Autodesk Fusion 360 part; units mm, degrees
note: some values were not read from the file. Chosen so that the rebuilt part matches the saved one: which bodies a step acts on. Set by a fixed rule: which sketch regions a step uses.
(part 2 of 2)
  measures "d487" distance of P900 P901
  measures "d488" distance of P898 P900
  measures "d489" radius of A29
  measures "d490" distance of P902 L38
  measures "d491" distance of P902 L39
  measures "d492" horizontal distance of P899 P902
  measures "d493" vertical distance of P899 P902
  measures "d603" distance of L42.start L42.end
  measures "d604" distance of L42.end L43.end
  measures "d608" diameter of A30
extrude "Extruir23" cut sketch "Boceto5" against normal blind 5 contours L8 L9 L10 L13 | L8 L9 L12 L13 | L8 L9 L11 L12 | L8 L9 L10 L11 | L8 L12 L42 L43 | L8 L12 L44 L45 bodies 10
extrude "Extruir24" add sketch "Boceto5" against normal blind 2 contours A4 | A5 | A6 | A7 bodies 10
extrude "Extruir61" cut sketch "Boceto5" against normal blind 7 contours L8 L47 L50 L51 L52 | L8 A30 L46 L47 L48 | A30 | A30 L46 L49 | A30 L48 L49 bodies 10
extrude "Extruir25" cut sketch "Boceto5" against normal blind 49 contours A8 | A9 bodies 10
extrude "Extruir26" add sketch "Boceto5" along normal blind 17 separate body contours A8 makes body 11
extrude "Extruir27" add sketch "Boceto5" along normal blind 14 separate body contours A9 makes body 12
extrude "Extruir28" cut sketch "Boceto5" along normal blind 4 contours A9 bodies 12
move_body "Desplazar2" bodies 11 12 to x (1, 0, 0) y (0, 1, 0) z (0, 0, 1) at (40.9619, 25.058, 2.4329)
combine "Combinar2" operation add target body 11 tool bodies 12
sketch "Boceto8" plane through (0, 0, 37) normal (0, 0, 1) x (1, 0, 0)
  arc A0 (-8.5, -7.5) -> (-7.5, -8.5) centre (-7.5, -7.5) ccw
  line L0 (-6, -6) -> (-6, 6)
  arc A1 (8.5, 7.5) -> (7.5, 8.5) centre (7.5, 7.5) ccw
  arc A2 (7.5, -8.5) -> (8.5, -7.5) centre (7.5, -7.5) ccw
  arc A3 (7.5, 6.5) -> (6.5, 7.5) centre (6.5, 6.5) ccw
  line L1 (-6, 6) -> (6, 6)
  line L2 (-7.5, -6.5) -> (-7.5, 6.5)
  line L3 (-7.5, 8.5) -> (7.5, 8.5)
  arc A4 (-6.5, 7.5) -> (-7.5, 6.5) centre (-6.5, 6.5) ccw
  line L4 (-8.5, -7.5) -> (-8.5, 7.5)
  line L5 (6.5, -7.5) -> (-6.5, -7.5)
  arc A5 (-7.5, 8.5) -> (-8.5, 7.5) centre (-7.5, 7.5) ccw
  circle A6 centre (0, 0) radius 1.5
  line L6 (-6.5, 7.5) -> (6.5, 7.5)
  line L7 (7.5, -8.5) -> (-7.5, -8.5)
  arc A7 (6.5, -7.5) -> (7.5, -6.5) centre (6.5, -6.5) ccw
  line L8 (8.5, 7.5) -> (8.5, -7.5)
  line L9 (6, 6) -> (6, -6)
  line L10 (7.5, 6.5) -> (7.5, -6.5)
  arc A8 (-7.5, -6.5) -> (-6.5, -7.5) centre (-6.5, -6.5) ccw
  line L11 (6, -6) -> (-6, -6)
  point P0 (7.5, 7.5)
  point P1 (-7.5, -7.5)
  point P2 (-7.5, 7.5)
  dimension "d241" = 1.5
  dimension "d242" = 15
  dimension "d243" = 15
  dimension "d244" = 1
  dimension "d245" = 1
  dimension "d246" = 1
  dimension "d247" = 1
  dimension "d248" = 1
  dimension "d249" = 1
  dimension "d250" = 1
  dimension "d251" = 1
  dimension "d252" = 1
  dimension "d253" = 7.5
  dimension "d254" = 7.5
  dimension "d255" = 3
  constraint horizontal L6
  constraint vertical L10
  constraint horizontal L5
  constraint vertical L2
  constraint tangent L4 A5
  constraint tangent L3 A5
  constraint tangent A0 L7
  constraint tangent A0 L4
  constraint equal A0 A5
  constraint tangent A2 L7
  constraint tangent A2 L8
  constraint equal A2 A5
  constraint tangent A1 L3
  constraint tangent A1 L8
  constraint equal A1 A5
  constraint coincident P2 L6
  constraint coincident P2 L2
  constraint tangent A4 L6
  constraint tangent L2 A4
  constraint coincident P0 L6
  constraint coincident P0 L10
  constraint tangent A3 L6
  constraint tangent A3 L10
  constraint tangent A7 L10
  constraint tangent L5 A7
  constraint coincident P1 L5
  constraint coincident P1 L2
  constraint tangent L5 A8
  constraint tangent L2 A8
  constraint coincident A6.centre origin
  measures "d242" distance of P0 P2
  measures "d243" distance of P1 P2
  measures "d244" distance of L5 L7
  measures "d245" distance of L2 L4
  measures "d246" distance of L3 L6
  measures "d247" distance of L8 L10
  measures "d248" radius of A5
  measures "d249" radius of A4
  measures "d250" radius of A3
  measures "d251" radius of A7
  measures "d252" radius of A8
  measures "d253" distance of A6.centre L2
  measures "d254" distance of A6.centre L6
  measures "d255" diameter of A6
extrude "Extruir32" add sketch "Boceto8" along normal blind 13 separate body contours L0 L1 L9 L11 | A6 makes body 13
extrude "Extruir34" add sketch "Boceto8" along normal blind 8 contours A3 L2 A4 L5 L6 A7 L10 A8 bodies 13
split "Dividir3" by plane through (0, 0, 45) normal (0, 0, 1) bodies 13 makes body 14 at (-2, 2, 50)
loft "Solevación1" add section 1 face at (-2, 2, 50) section 2 face at (-7, 2, 45) on bodies 13 14 bodies 13 14
extrude "Extruir35" cut sketch "Boceto8" along normal blind 7 contours A6 bodies 13
move_body "Desplazar14" bodies 13 to x (1, 0, 0) y (0, 1, 0) z (0, 0, 1) at (38.8109, 89.6933, 0)
copy_body "CopiarPegarCuerpos4" bodies 13 makes body 15
copy_body "CopiarPegarCuerpos5" bodies 13 makes body 16
move_body "Desplazar15" bodies 16 to x (1, 0, 0) y (0, 1, 0) z (0, 0, 1) at (59, 0, 0)
move_body "Desplazar16" bodies 15 to x (1, 0, 0) y (0, 1, 0) z (0, 0, 1) at (27, 0, 0)
copy_body "CopiarPegarCuerpos6" bodies 15 13 makes body 17 makes body 18
move_body "Desplazar17" bodies 17 18 to x (1, 0, 0) y (0, 1, 0) z (0, 0, 1) at (16.8789, 23.4733, 0)
extrude "Extruir38" cut sketch "Boceto5" against normal blind 2 contours L15 L30 A18 A19 L32 L33 A20 A21 | A10 L18 L19 L20 L21 A11 A12 A13 | L26 A14 L27 L28 A15 A16 A17 L29 | L34 A22 L35 A23 L36 L37 A24 A25 | L38 A26 L39 A27 L40 L41 A28 A29 bodies 10
move_body "Desplazar19" bodies 10 to x (-1, 0, 0) y (0, 1, 0) z (0, 0, -1) at (333, 0, 29)
move_body "Desplazar20" bodies 10 to x (1, 0, 0) y (0, -1, 0) z (0, 0, -1) at (-92.7675, 172.987, 0)
move_body "Desplazar21" bodies 10 to x (-1, 0, 0) y (0, -1, 0) z (0, 0, 1) at (125.3099, 172.9124, 50)
move_body "Desplazar22" bodies 10 to x (1, 0, 0) y (0, 1, 0) z (0, 0, 1) at (0, 0, -5)
move_body "Desplazar25" bodies 11 to x (1, 0, 0) y (0, 1, 0) z (0, 0, 1) at (-106.2292, 49.468, 0)
split "Dividir5" by plane through (50, 0, 6) normal (0, 0, 1) bodies 1 makes body 19 at (32.6667, 76, 13.3333)
combine "Combinar4" operation add target body 19 tool bodies 1
sketch "Boceto12" plane through (0, 76, 0) normal (0, 1, 0) x (-1, 0, 0)
  line L0 (2, 0) -> (2, 28)
  line L1 (2, 28) -> (-102, 28)
  line L2 (-102, 28) -> (-102, 0)
  line L3 (-102, 0) -> (2, 0)
  line L4 (2, 0) -> (-102, 0)
  line L5 (-18.3, 23.5) -> (-6.3, 23.5)
  line L6 (-6.3, 23.5) -> (-6.3, 17.5)
  line L7 (-6.3, 17.5) -> (-18.3, 17.5)
  line L8 (-18.3, 17.5) -> (-18.3, 23.5)
  line L9 (-0.55, 5) -> (-3.05, 5)
  point P0 (-120.95, 37)
  point P1 (-118.41, 37)
  point P2 (-1.8, 0)
  point P3 (-12.3, 17.5)
  point P4 (-115, 37)
  point P5 (-118.41, 37)
  point P6 (-136.19, 37)
  dimension "d590" = 12
  dimension "d591" = 6
  dimension "d594" = 12.5
  dimension "d616" = 17.78
  dimension "d617" = 3.41
  dimension "d619" = 12.3
  constraint horizontal L5
  constraint vertical L6
  constraint horizontal L7
  constraint vertical L8
  constraint midpoint L7 P3
  measures "d590" distance of L5.start L5.end
  measures "d591" distance of L5.start L7.end
  measures "d594" vertical distance of L6.end L9.end
  measures "d616" distance of P5 P6
  measures "d617" distance of P4 P5
  measures "d619" horizontal distance of origin P3
extrude "Extruir56" cut sketch "Boceto12" against normal blind 7 contours L5 L6 L7 L8 bodies 19
sketch "Boceto14" plane through (0, 73.9254, 0) normal (0, 1, 0) x (-1, 0, 0)
  line L0 (-102.0774, 44) -> (1.9226, 44)
  line L1 (1.9226, 44) -> (1.9226, 52)
  line L2 (1.9226, 52) -> (-102.0774, 52)
  line L3 (-102.0774, 52) -> (-102.0774, 44)
  line L4 (-20, 47.5) -> (-8, 47.5)
  line L5 (-8, 47.5) -> (-8, 41.5)
  line L6 (-8, 41.5) -> (-20, 41.5)
  line L7 (-20, 41.5) -> (-20, 47.5)
  line L8 (-18.3, 17.5) -> (-18.3, 23.5)
  line L9 (-18.3, 23.5) -> (-6.3, 23.5)
  line L10 (2, 28) -> (-102, 28)
  line L11 (-8, 47.5) -> (-20, 47.5)
  line L12 (-20, 47.5) -> (-20, 52)
  line L13 (-20, 52) -> (-8, 52)
  line L14 (-8, 52) -> (-8, 47.5)
  dimension "d595" = 6
  dimension "d596" = 12
  dimension "d597" = 12
  dimension "d598" = 6
  dimension "d599" = 4.5
  dimension "d600" = 4.5
  constraint horizontal L4
  constraint vertical L5
  constraint horizontal L6
  constraint vertical L7
  constraint horizontal L11
  constraint vertical L12
  constraint horizontal L13
  constraint vertical L14
  constraint coincident L2 L12.end
  measures "d595" distance of L8.start L8.end
  measures "d596" distance of L8.end L9.end
  measures "d597" distance of L4.start L4.end
  measures "d598" distance of L4.start L6.end
  measures "d599" distance of L9 L10
  measures "d600" distance of L2 L4
extrude "Extruir58" cut sketch "Boceto14" against normal blind 17 contours L0 L4 L5 L7 L11 | L0 L5 L6 L7 | L2 L4 L11 L12 L13 L14 bodies 10
hidden bodies 11 19 15 16 17 18
equation "d136 = ( ( 35.35 - 34.4 ) / 2 ) * 1 mm"
equation "d242 = d243"
equation "d253 = d254"
equation "d254 = d242 / 2"
equation "d282 = d23"
equation "d289 = d287"
equation "d291 = d287"
equation "d293 = ( d286 - d290 ) / 2"
equation "d294 = ( d285 / 2 - d292 ) / 2"
equation "d295 = d288"
equation "d296 = d288"
equation "d303 = d293"
equation "d308 = d294"
equation "d315 = d290"
equation "d316 = -d292"
equation "d323 = -d35 / 2"
equation "d328 = d323"
equation "d339 = d285"
equation "d341 = d286"
equation "d342 = d335"
equation "d343 = d336"
equation "d363 = d339 / 2"
equation "d385 = -17 * 0.1 in"
equation "d386 = 23 * 0.1 in"
equation "d387 = ( d363 - d388 ) / 2"
equation "d390 = ( d341 - d389 ) / 2"
equation "d398 = d243"
equation "d399 = d243"
equation "d436 = d243"
equation "d437 = d243"
equation "d438 = d248"
equation "d439 = d398 / 2"
equation "d440 = d399 / 2"
equation "d443 = d444 * 2"
equation "d445 = d444"
equation "d446 = d444"
equation "d449 = d448"
equation "d450 = d447"
equation "d451 = d447"
equation "d452 = d446"
equation "d453 = d443 / 2"
equation "d455 = d458 * 2 / 3"
equation "d460 = d455"
equation "d461 = d460"
equation "d464 = d243"
equation "d465 = d243"
equation "d466 = d248"
equation "d467 = d398 / 2"
equation "d468 = d399 / 2"
equation "d473 = d243"
equation "d474 = d243"
equation "d475 = d248"
equation "d476 = d398 / 2"
equation "d477 = d399 / 2"
equation "d480 = d243"
equation "d481 = d243"
equation "d482 = d248"
equation "d483 = d398 / 2"
equation "d484 = d399 / 2"
equation "d487 = d243"
equation "d488 = d243"
equation "d489 = d248"
equation "d490 = d398 / 2"
equation "d491 = d399 / 2"
equation "d594 = 18.5 mm - d591"
equation "d597 = d596"
equation "d598 = d595"
equation "d600 = d599"
equation "d603 = d127"
equation "d619 = d617 + d616 / 2"
named bodies: "Base", "Tapa", "Encoder", "Tecla", "Tecla (2)", "Tecla (2) (1)", "Tecla (3)", "Tecla (2) (1) (1)", "Tecla (2) (2)", "Tecla (4)", "Tecla (1)"
